Autodesk Inventor part; units mm, degrees
(part 15 of 16)
  spline S109 degree 3 poles (-20.4235, 24.8999) (-20.3314, 25.0779) (-20.2053, 25.3055) (-20.0401, 25.5749) (-19.9493, 25.7161) (-19.8616, 25.8465) (-19.7774, 25.9661) (-19.6971, 26.0752) (-19.6212, 26.174) (-19.55, 26.2628) (-19.4839, 26.3417) (-19.4233, 26.411) (-19.3686, 26.4711) (-19.3201, 26.5222) (-19.2781, 26.5645) (-19.2306, 26.6108) (-19.1862, 26.6499) (-19.1456, 26.6873) (-19.119, 26.7128) (-19.0934, 26.7382) (-19.0688, 26.7635) (-19.0454, 26.7887) (-19.0229, 26.8139) (-19.0014, 26.8391) (-18.9809, 26.8643) (-18.9614, 26.8898) (-18.9428, 26.9154) (-18.925, 26.9415) (-18.9082, 26.9681) (-18.8922, 26.9953) (-18.8771, 27.0236) (-18.863, 27.0531) (-18.8498, 27.0842) (-18.8379, 27.1174) (-18.8274, 27.1531) (-18.8189, 27.192) (-18.813, 27.2347) (-18.8107, 27.2815) (-18.8136, 27.3328) (-18.8231, 27.3881) (-18.8411, 27.4459) (-18.8673, 27.5015) (-18.9487, 27.622) (-19.0935, 27.7983) (-19.2204, 27.9879) (-19.3121, 28.1007) (-19.3578, 28.1419) (-19.4079, 28.1759) (-19.458, 28.201) (-19.5063, 28.2185) (-19.5518, 28.2299) (-19.5943, 28.2366) (-19.634, 28.2397) (-19.6713, 28.24) (-19.7065, 28.2382) (-19.7401, 28.2347) (-19.7724, 28.2296) (-19.8038, 28.2234) (-19.8346, 28.216) (-19.8649, 28.2076) (-19.8949, 28.1981) (-19.9249, 28.1877) (-19.9549, 28.1764) (-19.985, 28.1641) (-20.0153, 28.1508) (-20.046, 28.1366) (-20.0769, 28.1214) (-20.1082, 28.1053) (-20.1399, 28.0881) (-20.172, 28.07) (-20.2196, 28.042) (-20.2698, 28.0108) (-20.3279, 27.9787) (-20.3806, 27.9507) (-20.4435, 27.9191) (-20.5168, 27.8841) (-20.6008, 27.8462) (-20.6954, 27.8058) (-20.801, 27.7633) (-20.9175, 27.7192) (-21.0452, 27.674) (-21.1841, 27.628) (-21.3342, 27.5818) (-21.4957, 27.5358) (-21.8014, 27.4556) (-22.0557, 27.4007) (-22.2528, 27.3641) knots 0 0 0 0 0.085622 0.111078 0.134991 0.157361 0.178189 0.197474 0.215216 0.231415 0.246072 0.259186 0.270757 0.280785 0.28927 0.296213 0.309142 0.314525 0.319779 0.32491 0.329923 0.334826 0.339627 0.344336 0.348964 0.353525 0.358035 0.362514 0.366985 0.371475 0.37602 0.380661 0.385447 0.39044 0.395711 0.401345 0.407436 0.41408 0.421363 0.429333 0.437971 0.447155 0.455484 0.5 0.544516 0.552845 0.562029 0.570667 0.578637 0.58592 0.592564 0.598655 0.604289 0.60956 0.614553 0.619339 0.62398 0.628525 0.633015 0.637486 0.641965 0.646475 0.651036 0.655664 0.660373 0.665174 0.670077 0.67509 0.680221 0.685475 0.690858 0.703787 0.71073 0.719215 0.729243 0.740814 0.753928 0.768585 0.784784 0.802526 0.821811 0.842639 0.865009 0.888922 0.914378 1 1 1 1
  arc A314 (-20.4235, 24.8999) -> (-19.6884, 24.0568) centre (0.0409, 42.0024) ccw
  spline S110 degree 3 poles (-17.4962, 21.9091) (-17.4331, 22.0994) (-17.3441, 22.3438) (-17.223, 22.6357) (-17.1554, 22.7895) (-17.0892, 22.932) (-17.0247, 23.0633) (-16.9626, 23.1836) (-16.903, 23.2931) (-16.8466, 23.3918) (-16.7937, 23.4801) (-16.7447, 23.5581) (-16.7, 23.626) (-16.6601, 23.684) (-16.6253, 23.7324) (-16.5855, 23.7856) (-16.5478, 23.8311) (-16.5136, 23.8744) (-16.4912, 23.9038) (-16.4699, 23.9329) (-16.4497, 23.9617) (-16.4304, 23.9902) (-16.4122, 24.0186) (-16.3949, 24.0469) (-16.3786, 24.075) (-16.3633, 24.1032) (-16.3489, 24.1315) (-16.3355, 24.16) (-16.323, 24.1889) (-16.3115, 24.2183) (-16.301, 24.2486) (-16.2916, 24.2799) (-16.2835, 24.3127) (-16.2769, 24.3473) (-16.2722, 24.3843) (-16.2698, 24.424) (-16.2707, 24.4671) (-16.2758, 24.5137) (-16.2866, 24.5639) (-16.3047, 24.617) (-16.3315, 24.6713) (-16.3661, 24.7221) (-16.4653, 24.8284) (-16.636, 24.9798) (-16.7909, 25.1473) (-16.8991, 25.2444) (-16.9507, 25.2779) (-17.0055, 25.3036) (-17.0589, 25.3206) (-17.1094, 25.3304) (-17.1561, 25.3345) (-17.1992, 25.3345) (-17.2389, 25.3313) (-17.2757, 25.3258) (-17.3102, 25.3185) (-17.3428, 25.3097) (-17.3739, 25.2997) (-17.404, 25.2886) (-17.4332, 25.2765) (-17.4618, 25.2634) (-17.49, 25.2494) (-17.518, 25.2345) (-17.5459, 25.2185) (-17.5737, 25.2017) (-17.6016, 25.1838) (-17.6296, 25.165) (-17.6577, 25.1452) (-17.6861, 25.1243) (-17.7148, 25.1024) (-17.7437, 25.0795) (-17.7863, 25.0444) (-17.831, 25.0058) (-17.8834, 24.9649) (-17.931, 24.9291) (-17.9882, 24.888) (-18.0551, 24.842) (-18.1321, 24.7914) (-18.2193, 24.7367) (-18.3169, 24.6782) (-18.4251, 24.6165) (-18.5441, 24.5518) (-18.6741, 24.4847) (-18.8152, 24.4156) (-18.9675, 24.3448) (-19.2569, 24.2178) (-19.4995, 24.1238) (-19.6884, 24.0568) knots 0 0 0 0 0.085622 0.111078 0.134991 0.157361 0.178189 0.197474 0.215216 0.231415 0.246072 0.259186 0.270757 0.280785 0.28927 0.296213 0.309142 0.314525 0.319779 0.32491 0.329923 0.334826 0.339627 0.344336 0.348964 0.353525 0.358035 0.362514 0.366985 0.371475 0.37602 0.380661 0.385447 0.39044 0.395711 0.401345 0.407436 0.41408 0.421363 0.429333 0.437971 0.447155 0.455484 0.5 0.544516 0.552845 0.562029 0.570667 0.578637 0.58592 0.592564 0.598655 0.604289 0.60956 0.614553 0.619339 0.62398 0.628525 0.633015 0.637486 0.641965 0.646475 0.651036 0.655664 0.660373 0.665174 0.670077 0.67509 0.680221 0.685475 0.690858 0.703787 0.71073 0.719215 0.729243 0.740814 0.753928 0.768585 0.784784 0.802526 0.821811 0.842639 0.865009 0.888922 0.914378 1 1 1 1
  arc A315 (-17.4962, 21.9091) -> (-16.6382, 21.1914) centre (0.0409, 42.0024) ccw
  spline S111 degree 3 poles (-14.137, 19.4131) (-14.1044, 19.6109) (-14.0548, 19.8663) (-13.9809, 20.1735) (-13.9381, 20.3359) (-13.895, 20.487) (-13.8519, 20.6268) (-13.8093, 20.7554) (-13.7676, 20.8728) (-13.7273, 20.9792) (-13.6889, 21.0747) (-13.6527, 21.1594) (-13.6192, 21.2334) (-13.5889, 21.297) (-13.562, 21.3502) (-13.5311, 21.4089) (-13.5009, 21.4598) (-13.4739, 21.5079) (-13.4565, 21.5404) (-13.44, 21.5725) (-13.4245, 21.6041) (-13.4099, 21.6353) (-13.3963, 21.6662) (-13.3837, 21.6968) (-13.372, 21.7272) (-13.3613, 21.7574) (-13.3515, 21.7876) (-13.3427, 21.8178) (-13.3349, 21.8483) (-13.3281, 21.8792) (-13.3225, 21.9107) (-13.3182, 21.9431) (-13.3153, 21.9768) (-13.3142, 22.012) (-13.3153, 22.0493) (-13.3192, 22.0889) (-13.3267, 22.1313) (-13.3391, 22.1765) (-13.3576, 22.2244) (-13.3837, 22.2741) (-13.4187, 22.3235) (-13.4608, 22.3683) (-13.5755, 22.4577) (-13.7677, 22.5806) (-13.9469, 22.7218) (-14.069, 22.8007) (-14.1252, 22.8258) (-14.1834, 22.8426) (-14.2388, 22.851) (-14.2901, 22.8527) (-14.337, 22.8495) (-14.3795, 22.8427) (-14.4182, 22.8334) (-14.4537, 22.8222) (-14.4866, 22.8096) (-14.5175, 22.7958) (-14.5467, 22.7811) (-14.5746, 22.7654) (-14.6016, 22.7489) (-14.6278, 22.7315) (-14.6535, 22.7132) (-14.6787, 22.6941) (-14.7038, 22.674) (-14.7286, 22.653) (-14.7533, 22.631) (-14.7781, 22.608) (-14.8028, 22.5841) (-14.8276, 22.559) (-14.8524, 22.5329) (-14.8774, 22.5057) (-14.914, 22.4644) (-14.9521, 22.4192) (-14.9974, 22.3707) (-15.0389, 22.3279) (-15.0889, 22.2784) (-15.1479, 22.2224) (-15.216, 22.1604) (-15.2935, 22.0927) (-15.3808, 22.0197) (-15.478, 21.9418) (-15.5855, 21.8593) (-15.7033, 21.7727) (-15.8319, 21.6823) (-15.9712, 21.5886) (-16.2372, 21.4179) (-16.4621, 21.2871) (-16.6382, 21.1914) knots 0 0 0 0 0.085622 0.111078 0.134991 0.157361 0.178189 0.197474 0.215216 0.231415 0.246072 0.259186 0.270757 0.280785 0.28927 0.296213 0.309142 0.314525 0.319779 0.32491 0.329923 0.334826 0.339627 0.344336 0.348964 0.353525 0.358035 0.362514 0.366985 0.371475 0.37602 0.380661 0.385447 0.39044 0.395711 0.401345 0.407436 0.41408 0.421363 0.429333 0.437971 0.447155 0.455484 0.5 0.544516 0.552845 0.562029 0.570667 0.578637 0.58592 0.592564 0.598655 0.604289 0.60956 0.614553 0.619339 0.62398 0.628525 0.633015 0.637486 0.641965 0.646475 0.651036 0.655664 0.660373 0.665174 0.670077 0.67509 0.680221 0.685475 0.690858 0.703787 0.71073 0.719215 0.729243 0.740814 0.753928 0.768585 0.784784 0.802526 0.821811 0.842639 0.865009 0.888922 0.914378 1 1 1 1
  arc A316 (-14.137, 19.4131) -> (-13.1773, 18.8385) centre (0.0409, 42.0024) ccw
  spline S112 degree 3 poles (-10.4287, 17.4733) (-10.4274, 17.6737) (-10.4184, 17.9337) (-10.3934, 18.2488) (-10.3767, 18.4159) (-10.3577, 18.5718) (-10.337, 18.7166) (-10.315, 18.8503) (-10.2922, 18.9728) (-10.2691, 19.0842) (-10.246, 19.1845) (-10.2235, 19.2738) (-10.2021, 19.3522) (-10.182, 19.4197) (-10.1638, 19.4765) (-10.1425, 19.5393) (-10.1206, 19.5943) (-10.1015, 19.646) (-10.0893, 19.6809) (-10.0781, 19.7151) (-10.0677, 19.7488) (-10.0582, 19.7819) (-10.0496, 19.8145) (-10.0419, 19.8467) (-10.0351, 19.8785) (-10.0293, 19.9101) (-10.0243, 19.9414) (-10.0203, 19.9727) (-10.0174, 20.004) (-10.0156, 20.0356) (-10.0149, 20.0676) (-10.0157, 20.1003) (-10.0182, 20.134) (-10.0226, 20.1689) (-10.0295, 20.2055) (-10.0395, 20.2441) (-10.0536, 20.2847) (-10.0729, 20.3275) (-10.0987, 20.372) (-10.1323, 20.4169) (-10.1745, 20.4602) (-10.2232, 20.4979) (-10.3504, 20.5682) (-10.5595, 20.6596) (-10.7586, 20.771) (-10.8915, 20.8298) (-10.9509, 20.8458) (-11.011, 20.8533) (-11.0671, 20.8529) (-11.118, 20.8466) (-11.1638, 20.8361) (-11.2047, 20.8228) (-11.2415, 20.8075) (-11.2748, 20.7909) (-11.3053, 20.7733) (-11.3337, 20.7549) (-11.3602, 20.7357) (-11.3853, 20.7159) (-11.4094, 20.6953) (-11.4325, 20.6741) (-11.4551, 20.652) (-11.477, 20.6291) (-11.4986, 20.6054) (-11.5199, 20.5808) (-11.5409, 20.5552) (-11.5617, 20.5286) (-11.5823, 20.5011) (-11.6029, 20.4725) (-11.6234, 20.4428) (-11.6438, 20.412) (-11.6734, 20.3655) (-11.704, 20.3149) (-11.7412, 20.2599) (-11.7754, 20.2111) (-11.8171, 20.1544) (-11.8666, 20.0899) (-11.9242, 20.018) (-11.9902, 19.939) (-12.065, 19.8533) (-12.1488, 19.7611) (-12.242, 19.6628) (-12.3449, 19.5588) (-12.4577, 19.4495) (-12.5807, 19.3351) (-12.8166, 19.1249) (-13.0183, 18.9605) (-13.1773, 18.8385) knots 0 0 0 0 0.085622 0.111078 0.134991 0.157361 0.178189 0.197474 0.215216 0.231415 0.246072 0.259186 0.270757 0.280785 0.28927 0.296213 0.309142 0.314525 0.319779 0.32491 0.329923 0.334826 0.339627 0.344336 0.348964 0.353525 0.358035 0.362514 0.366985 0.371475 0.37602 0.380661 0.385447 0.39044 0.395711 0.401345 0.407436 0.41408 0.421363 0.429333 0.437971 0.447155 0.455484 0.5 0.544516 0.552845 0.562029 0.570667 0.578637 0.58592 0.592564 0.598655 0.604289 0.60956 0.614553 0.619339 0.62398 0.628525 0.633015 0.637486 0.641965 0.646475 0.651036 0.655664 0.660373 0.665174 0.670077 0.67509 0.680221 0.685475 0.690858 0.703787 0.71073 0.719215 0.729243 0.740814 0.753928 0.768585 0.784784 0.802526 0.821811 0.842639 0.865009 0.888922 0.914378 1 1 1 1
  arc A317 (-10.4287, 17.4733) -> (-9.3909, 17.0559) centre (0.0409, 42.0024) ccw
  spline S113 degree 3 poles (-6.4626, 16.1375) (-6.4927, 16.3356) (-6.5245, 16.5939) (-6.5491, 16.9089) (-6.5587, 17.0766) (-6.5643, 17.2336) (-6.5665, 17.3799) (-6.5657, 17.5153) (-6.5624, 17.6399) (-6.557, 17.7535) (-6.5499, 17.8562) (-6.5416, 17.9479) (-6.5327, 18.0287) (-6.5235, 18.0985) (-6.5144, 18.1574) (-6.5031, 18.2228) (-6.4901, 18.2805) (-6.4793, 18.3346) (-6.4728, 18.371) (-6.467, 18.4065) (-6.462, 18.4414) (-6.4578, 18.4756) (-6.4545, 18.5092) (-6.4519, 18.5422) (-6.4502, 18.5747) (-6.4493, 18.6067) (-6.4493, 18.6385) (-6.4503, 18.67) (-6.4523, 18.7014) (-6.4554, 18.7328) (-6.4598, 18.7646) (-6.4657, 18.7967) (-6.4733, 18.8296) (-6.4832, 18.8635) (-6.4957, 18.8985) (-6.5117, 18.935) (-6.532, 18.973) (-6.5577, 19.0122) (-6.5901, 19.0521) (-6.6303, 19.0912) (-6.6788, 19.1274) (-6.7327, 19.157) (-6.8694, 19.2066) (-7.0902, 19.2641) (-7.3043, 19.3429) (-7.4448, 19.3803) (-7.506, 19.3868) (-7.5665, 19.3848) (-7.6218, 19.3756) (-7.6712, 19.3614) (-7.7147, 19.3439) (-7.753, 19.3243) (-7.787, 19.3035) (-7.8173, 19.2819) (-7.8447, 19.2597) (-7.8698, 19.2371) (-7.893, 19.214) (-7.9147, 19.1905) (-7.9352, 19.1665) (-7.9548, 19.1418) (-7.9736, 19.1165) (-7.9917, 19.0905) (-8.0093, 19.0637) (-8.0264, 19.036) (-8.0432, 19.0074) (-8.0596, 18.978) (-8.0757, 18.9475) (-8.0915, 18.916) (-8.1071, 18.8835) (-8.1224, 18.85) (-8.1445, 18.7994) (-8.1668, 18.7446) (-8.1949, 18.6845) (-8.2211, 18.6309) (-8.2534, 18.5683) (-8.2921, 18.4969) (-8.3377, 18.4169) (-8.3906, 18.3286) (-8.451, 18.2322) (-8.5194, 18.128) (-8.5961, 18.0164) (-8.6814, 17.8976) (-8.7757, 17.7719) (-8.8794, 17.6397) (-9.0795, 17.3952) (-9.253, 17.2013) (-9.3909, 17.0559) knots 0 0 0 0 0.085622 0.111078 0.134991 0.157361 0.178189 0.197474 0.215216 0.231415 0.246072 0.259186 0.270757 0.280785 0.28927 0.296213 0.309142 0.314525 0.319779 0.32491 0.329923 0.334826 0.339627 0.344336 0.348964 0.353525 0.358035 0.362514 0.366985 0.371475 0.37602 0.380661 0.385447 0.39044 0.395711 0.401345 0.407436 0.41408 0.421363 0.429333 0.437971 0.447155 0.455484 0.5 0.544516 0.552845 0.562029 0.570667 0.578637 0.58592 0.592564 0.598655 0.604289 0.60956 0.614553 0.619339 0.62398 0.628525 0.633015 0.637486 0.641965 0.646475 0.651036 0.655664 0.660373 0.665174 0.670077 0.67509 0.680221 0.685475 0.690858 0.703787 0.71073 0.719215 0.729243 0.740814 0.753928 0.768585 0.784784 0.802526 0.821811 0.842639 0.865009 0.888922 0.914378 1 1 1 1
  arc A318 (-6.4626, 16.1375) -> (-5.3723, 15.8875) centre (0.0409, 42.0024) ccw
  spline S114 degree 3 poles (-2.3363, 15.4385) (-2.3971, 15.6296) (-2.4689, 15.8796) (-2.5425, 16.187) (-2.5782, 16.3511) (-2.6083, 16.5053) (-2.6334, 16.6494) (-2.6538, 16.7833) (-2.67, 16.9068) (-2.6824, 17.0199) (-2.6914, 17.1225) (-2.6977, 17.2143) (-2.7014, 17.2955) (-2.7032, 17.3659) (-2.7035, 17.4255) (-2.7026, 17.4919) (-2.6988, 17.5509) (-2.6966, 17.606) (-2.6958, 17.6429) (-2.6956, 17.679) (-2.6962, 17.7142) (-2.6974, 17.7486) (-2.6993, 17.7823) (-2.702, 17.8153) (-2.7053, 17.8477) (-2.7095, 17.8795) (-2.7145, 17.9108) (-2.7204, 17.9418) (-2.7272, 17.9725) (-2.7352, 18.0031) (-2.7445, 18.0337) (-2.7554, 18.0646) (-2.7681, 18.0959) (-2.7831, 18.1278) (-2.801, 18.1604) (-2.8225, 18.194) (-2.8484, 18.2283) (-2.88, 18.263) (-2.9183, 18.2973) (-2.9641, 18.3297) (-3.0177, 18.3578) (-3.0755, 18.3786) (-3.2183, 18.4062) (-3.4454, 18.4284) (-3.6691, 18.4729) (-3.8138, 18.4878) (-3.8752, 18.4846) (-3.9346, 18.4732) (-3.9879, 18.4555) (-4.0344, 18.4338) (-4.0746, 18.4096) (-4.1094, 18.3843) (-4.1397, 18.3584) (-4.1663, 18.3323) (-4.1899, 18.3061) (-4.2111, 18.2799) (-4.2304, 18.2535) (-4.2482, 18.2268) (-4.2647, 18.1999) (-4.2802, 18.1725) (-4.2948, 18.1445) (-4.3086, 18.116) (-4.3218, 18.0867) (-4.3344, 18.0567) (-4.3465, 18.0259) (-4.358, 17.9942) (-4.3692, 17.9616) (-4.3799, 17.9281) (-4.3902, 17.8935) (-4.4001, 17.858) (-4.4139, 17.8046) (-4.4274, 17.747) (-4.4458, 17.6832) (-4.4632, 17.6262) (-4.4854, 17.5593) (-4.5125, 17.4827) (-4.545, 17.3966) (-4.5834, 17.3011) (-4.628, 17.1964) (-4.6792, 17.0828) (-4.7375, 16.9606) (-4.8032, 16.8299) (-4.8767, 16.691) (-4.9584, 16.5442) (-5.1178, 16.2714) (-5.2588, 16.0528) (-5.3723, 15.8875) knots 0 0 0 0 0.085622 0.111078 0.134991 0.157361 0.178189 0.197474 0.215216 0.231415 0.246072 0.259186 0.270757 0.280785 0.28927 0.296213 0.309142 0.314525 0.319779 0.32491 0.329923 0.334826 0.339627 0.344336 0.348964 0.353525 0.358035 0.362514 0.366985 0.371475 0.37602 0.380661 0.385447 0.39044 0.395711 0.401345 0.407436 0.41408 0.421363 0.429333 0.437971 0.447155 0.455484 0.5 0.544516 0.552845 0.562029 0.570667 0.578637 0.58592 0.592564 0.598655 0.604289 0.60956 0.614553 0.619339 0.62398 0.628525 0.633015 0.637486 0.641965 0.646475 0.651036 0.655664 0.660373 0.665174 0.670077 0.67509 0.680221 0.685475 0.690858 0.703787 0.71073 0.719215 0.729243 0.740814 0.753928 0.768585 0.784784 0.802526 0.821811 0.842639 0.865009 0.888922 0.914378 1 1 1 1
  arc A319 (-2.3363, 15.4385) -> (-1.2204, 15.3622) centre (0.0409, 42.0024) ccw
  spline S115 degree 3 poles (1.8484, 15.3937) (1.7585, 15.5729) (1.6485, 15.8086) (1.5278, 16.1007) (1.4668, 16.2572) (1.4129, 16.4048) (1.3656, 16.5432) (1.3245, 16.6722) (1.2892, 16.7917) (1.2593, 16.9015) (1.2343, 17.0013) (1.2138, 17.0911) (1.1973, 17.1707) (1.1845, 17.24) (1.175, 17.2988) (1.1655, 17.3645) (1.16, 17.4234) (1.1535, 17.4782) (1.1486, 17.5147) (1.1431, 17.5504) (1.137, 17.5851) (1.1304, 17.6189) (1.1233, 17.6519) (1.1155, 17.684) (1.1071, 17.7155) (1.098, 17.7462) (1.0882, 17.7764) (1.0775, 17.806) (1.066, 17.8353) (1.0533, 17.8643) (1.0393, 17.8931) (1.0237, 17.9219) (1.0063, 17.9508) (0.9865, 17.9799) (0.9637, 18.0094) (0.9372, 18.0392) (0.9062, 18.069) (0.8696, 18.0984) (0.8265, 18.1263) (0.7762, 18.151) (0.7188, 18.1704) (0.6584, 18.1819) (0.5131, 18.1869) (0.2853, 18.1733) (0.0574, 18.1822) (-0.0878, 18.1743) (-0.148, 18.1616) (-0.2049, 18.141) (-0.2547, 18.1152) (-0.2973, 18.0864) (-0.3333, 18.0563) (-0.3637, 18.0258) (-0.3895, 17.9955) (-0.4117, 17.9656) (-0.4309, 17.936) (-0.4477, 17.9068) (-0.4627, 17.8777) (-0.4761, 17.8486) (-0.4882, 17.8194) (-0.4992, 17.7899) (-0.5092, 17.76) (-0.5184, 17.7296) (-0.5268, 17.6987) (-0.5346, 17.6671) (-0.5417, 17.6348) (-0.5482, 17.6017) (-0.5541, 17.5677) (-0.5594, 17.5329) (-0.5642, 17.4972) (-0.5684, 17.4605) (-0.5737, 17.4056) (-0.578, 17.3466) (-0.5862, 17.2807) (-0.5945, 17.2217) (-0.6059, 17.1522) (-0.6207, 17.0723) (-0.6393, 16.9821) (-0.6623, 16.8818) (-0.69, 16.7714) (-0.7229, 16.6512) (-0.7613, 16.5214) (-0.8057, 16.382) (-0.8566, 16.2333) (-0.9143, 16.0756) (-1.0291, 15.7812) (-1.1342, 15.5432) (-1.2204, 15.3622) knots 0 0 0 0 0.085622 0.111078 0.134991 0.157361 0.178189 0.197474 0.215216 0.231415 0.246072 0.259186 0.270757 0.280785 0.28927 0.296213 0.309142 0.314525 0.319779 0.32491 0.329923 0.334826 0.339627 0.344336 0.348964 0.353525 0.358035 0.362514 0.366985 0.371475 0.37602 0.380661 0.385447 0.39044 0.395711 0.401345 0.407436 0.41408 0.421363 0.429333 0.437971 0.447155 0.455484 0.5 0.544516 0.552845 0.562029 0.570667 0.578637 0.58592 0.592564 0.598655 0.604289 0.60956 0.614553 0.619339 0.62398 0.628525 0.633015 0.637486 0.641965 0.646475 0.651036 0.655664 0.660373 0.665174 0.670077 0.67509 0.680221 0.685475 0.690858 0.703787 0.71073 0.719215 0.729243 0.740814 0.753928 0.768585 0.784784 0.802526 0.821811 0.842639 0.865009 0.888922 0.914378 1 1 1 1
  arc A320 (1.8484, 15.3937) -> (2.9626, 15.4929) centre (0.0409, 42.0024) ccw
  spline S116 degree 3 poles (5.9887, 16.0041) (5.8719, 16.1669) (5.7263, 16.3826) (5.5614, 16.6522) (5.4767, 16.7972) (5.4004, 16.9345) (5.332, 17.0638) (5.2713, 17.1849) (5.2177, 17.2974) (5.1709, 17.4011) (5.1306, 17.4958) (5.0963, 17.5813) (5.0676, 17.6573) (5.0441, 17.7237) (5.0255, 17.7803) (5.0058, 17.8437) (4.9912, 17.901) (4.9763, 17.9541) (4.9656, 17.9895) (4.9546, 18.0238) (4.9432, 18.0572) (4.9314, 18.0895) (4.9192, 18.121) (4.9065, 18.1515) (4.8933, 18.1813) (4.8795, 18.2102) (4.8651, 18.2385) (4.8499, 18.2661) (4.8339, 18.2932) (4.8168, 18.3198) (4.7985, 18.3461) (4.7786, 18.3721) (4.7569, 18.3979) (4.7328, 18.4236) (4.7057, 18.4491) (4.6749, 18.4744) (4.6396, 18.499) (4.5988, 18.5223) (4.5518, 18.5431) (4.4983, 18.5597) (4.4386, 18.5699) (4.3771, 18.5718) (4.2328, 18.5539) (4.01, 18.5049) (3.7835, 18.478) (3.6413, 18.4475) (3.5839, 18.4255) (3.5309, 18.3963) (3.4857, 18.363) (3.4482, 18.328) (3.4173, 18.2926) (3.3921, 18.2577) (3.3713, 18.2237) (3.3541, 18.1907) (3.3397, 18.1585) (3.3277, 18.127) (3.3175, 18.0959) (3.3088, 18.0651) (3.3014, 18.0343) (3.2952, 18.0035) (3.2899, 17.9724) (3.2856, 17.941) (3.2821, 17.9091) (3.2794, 17.8767) (3.2774, 17.8436) (3.2762, 17.8099) (3.2757, 17.7755) (3.2758, 17.7402) (3.2767, 17.7042) (3.2783, 17.6673) (3.2816, 17.6123) (3.2866, 17.5533) (3.2889, 17.487) (3.2899, 17.4274) (3.2895, 17.357) (3.2874, 17.2757) (3.2831, 17.1837) (3.2761, 17.081) (3.266, 16.9677) (3.2523, 16.8439) (3.2347, 16.7096) (3.2126, 16.565) (3.1856, 16.4102) (3.1533, 16.2454) (3.086, 15.9366) (3.0194, 15.6851) (2.9626, 15.4929) knots 0 0 0 0 0.085622 0.111078 0.134991 0.157361 0.178189 0.197474 0.215216 0.231415 0.246072 0.259186 0.270757 0.280785 0.28927 0.296213 0.309142 0.314525 0.319779 0.32491 0.329923 0.334826 0.339627 0.344336 0.348964 0.353525 0.358035 0.362514 0.366985 0.371475 0.37602 0.380661 0.385447 0.39044 0.395711 0.401345 0.407436 0.41408 0.421363 0.429333 0.437971 0.447155 0.455484 0.5 0.544516 0.552845 0.562029 0.570667 0.578637 0.58592 0.592564 0.598655 0.604289 0.60956 0.614553 0.619339 0.62398 0.628525 0.633015 0.637486 0.641965 0.646475 0.651036 0.655664 0.660373 0.665174 0.670077 0.67509 0.680221 0.685475 0.690858 0.703787 0.71073 0.719215 0.729243 0.740814 0.753928 0.768585 0.784784 0.802526 0.821811 0.842639 0.865009 0.888922 0.914378 1 1 1 1
  arc A321 (5.9887, 16.0041) -> (7.0736, 16.2763) centre (0.0409, 42.0024) ccw
  spline S117 degree 3 poles (9.9825, 17.2546) (9.8416, 17.3972) (9.6642, 17.5874) (9.4591, 17.8278) (9.3528, 17.9579) (9.2559, 18.0816) (9.1681, 18.1986) (9.0892, 18.3086) (9.0187, 18.4114) (8.9563, 18.5065) (8.9016, 18.5937) (8.8544, 18.6728) (8.8142, 18.7434) (8.7806, 18.8053) (8.7533, 18.8583) (8.724, 18.9179) (8.7005, 18.9722) (8.6775, 19.0223) (8.6614, 19.0555) (8.6452, 19.0877) (8.6287, 19.1189) (8.612, 19.149) (8.595, 19.1781) (8.5777, 19.2063) (8.56, 19.2336) (8.5418, 19.2601) (8.5232, 19.2857) (8.5039, 19.3106) (8.4838, 19.3349) (8.4628, 19.3585) (8.4406, 19.3816) (8.4169, 19.4042) (8.3914, 19.4263) (8.3635, 19.4479) (8.3328, 19.4689) (8.2984, 19.489) (8.2597, 19.5078) (8.2158, 19.5244) (8.1662, 19.5376) (8.1107, 19.5456) (8.0501, 19.5464) (7.9891, 19.5386) (7.8494, 19.4984) (7.637, 19.4151) (7.4174, 19.3531) (7.2818, 19.3007) (7.2285, 19.27) (7.1807, 19.2329) (7.1413, 19.1929) (7.1097, 19.1524) (7.0848, 19.1127) (7.0653, 19.0743) (7.0501, 19.0375) (7.0383, 19.0022) (7.0291, 18.9681) (7.0221, 18.9351) (7.0169, 18.9028) (7.0132, 18.871) (7.0107, 18.8395) (7.0093, 18.808) (7.009, 18.7765) (7.0097, 18.7448) (7.0112, 18.7128) (7.0136, 18.6803) (7.0168, 18.6474) (7.0209, 18.6139) (7.0258, 18.5798) (7.0315, 18.545) (7.038, 18.5096) (7.0453, 18.4734) (7.0572, 18.4195) (7.0713, 18.3621) (7.084, 18.2969) (7.0942, 18.2382) (7.1049, 18.1686) (7.1155, 18.088) (7.1256, 17.9965) (7.1348, 17.894) (7.1426, 17.7805) (7.1485, 17.656) (7.152, 17.5206) (7.1528, 17.3743) (7.1504, 17.2172) (7.1443, 17.0494) (7.1261, 16.7339) (7.0997, 16.4751) (7.0736, 16.2763) knots 0 0 0 0 0.085622 0.111078 0.134991 0.157361 0.178189 0.197474 0.215216 0.231415 0.246072 0.259186 0.270757 0.280785 0.28927 0.296213 0.309142 0.314525 0.319779 0.32491 0.329923 0.334826 0.339627 0.344336 0.348964 0.353525 0.358035 0.362514 0.366985 0.371475 0.37602 0.380661 0.385447 0.39044 0.395711 0.401345 0.407436 0.41408 0.421363 0.429333 0.437971 0.447155 0.455484 0.5 0.544516 0.552845 0.562029 0.570667 0.578637 0.58592 0.592564 0.598655 0.604289 0.60956 0.614553 0.619339 0.62398 0.628525 0.633015 0.637486 0.641965 0.646475 0.651036 0.655664 0.660373 0.665174 0.670077 0.67509 0.680221 0.685475 0.690858 0.703787 0.71073 0.719215 0.729243 0.740814 0.753928 0.768585 0.784784 0.802526 0.821811 0.842639 0.865009 0.888922 0.914378 1 1 1 1
  arc A322 (9.9825, 17.2546) -> (11.0115, 17.6932) centre (0.0409, 42.0024) ccw
  spline S118 degree 3 poles (13.7315, 19.1145) (13.5701, 19.2333) (13.365, 19.3934) (13.1248, 19.5988) (12.9995, 19.7106) (12.8845, 19.8176) (12.7795, 19.9195) (12.6843, 20.0158) (12.5986, 20.1062) (12.5221, 20.1904) (12.4544, 20.2681) (12.3954, 20.3388) (12.3446, 20.4022) (12.3018, 20.4581) (12.2666, 20.5062) (12.2283, 20.5604) (12.1966, 20.6104) (12.166, 20.6563) (12.145, 20.6866) (12.1239, 20.7158) (12.1028, 20.744) (12.0815, 20.7712) (12.0602, 20.7973) (12.0387, 20.8224) (12.0169, 20.8466) (11.9949, 20.8699) (11.9724, 20.8923) (11.9495, 20.9139) (11.9259, 20.9347) (11.9014, 20.9548) (11.8759, 20.9741) (11.8489, 20.9927) (11.8203, 21.0105) (11.7894, 21.0275) (11.7557, 21.0434) (11.7186, 21.0579) (11.6774, 21.0704) (11.6315, 21.08) (11.5804, 21.0852) (11.5243, 21.0845) (11.4644, 21.0757) (11.4054, 21.0585) (11.2736, 20.997) (11.0769, 20.8815) (10.8697, 20.7859) (10.7439, 20.7129) (10.6961, 20.6743) (10.6547, 20.6301) (10.6221, 20.5845) (10.5972, 20.5396) (10.5788, 20.4964) (10.5656, 20.4554) (10.5563, 20.4167) (10.5502, 20.38) (10.5464, 20.3449) (10.5447, 20.3112) (10.5446, 20.2785) (10.5459, 20.2465) (10.5484, 20.215) (10.552, 20.1837) (10.5566, 20.1525) (10.5622, 20.1213) (10.5687, 20.0899) (10.5761, 20.0582) (10.5845, 20.0262) (10.5937, 19.9937) (10.6039, 19.9608) (10.6149, 19.9274) (10.6269, 19.8934) (10.6398, 19.8588) (10.66, 19.8074) (10.6829, 19.7529) (10.7056, 19.6905) (10.7249, 19.6342) (10.7463, 19.5671) (10.7694, 19.4892) (10.7938, 19.4003) (10.8189, 19.3005) (10.8443, 19.1896) (10.8696, 19.0676) (10.8943, 18.9344) (10.918, 18.7901) (10.9401, 18.6345) (10.9603, 18.4678) (10.9918, 18.1534) (11.0061, 17.8936) (11.0115, 17.6932) knots 0 0 0 0 0.085622 0.111078 0.134991 0.157361 0.178189 0.197474 0.215216 0.231415 0.246072 0.259186 0.270757 0.280785 0.28927 0.296213 0.309142 0.314525 0.319779 0.32491 0.329923 0.334826 0.339627 0.344336 0.348964 0.353525 0.358035 0.362514 0.366985 0.371475 0.37602 0.380661 0.385447 0.39044 0.395711 0.401345 0.407436 0.41408 0.421363 0.429333 0.437971 0.447155 0.455484 0.5 0.544516 0.552845 0.562029 0.570667 0.578637 0.58592 0.592564 0.598655 0.604289 0.60956 0.614553 0.619339 0.62398 0.628525 0.633015 0.637486 0.641965 0.646475 0.651036 0.655664 0.660373 0.665174 0.670077 0.67509 0.680221 0.685475 0.690858 0.703787 0.71073 0.719215 0.729243 0.740814 0.753928 0.768585 0.784784 0.802526 0.821811 0.842639 0.865009 0.888922 0.914378 1 1 1 1
  arc A323 (13.7315, 19.1145) -> (14.6792, 19.7087) centre (0.0409, 42.0024) ccw
  spline S119 degree 3 poles (17.1434, 21.5379) (16.9654, 21.63) (16.7378, 21.7561) (16.4684, 21.9214) (16.3272, 22.0122) (16.1968, 22.0999) (16.0772, 22.1841) (15.9681, 22.2644) (15.8693, 22.3403) (15.7805, 22.4115) (15.7016, 22.4776) (15.6322, 22.5381) (15.5722, 22.5929) (15.5211, 22.6414) (15.4788, 22.6833) (15.4325, 22.7309) (15.3934, 22.7753) (15.356, 22.8159) (15.3305, 22.8425) (15.3051, 22.8681) (15.2798, 22.8926) (15.2546, 22.9161) (15.2294, 22.9386) (15.2042, 22.96) (15.179, 22.9805) (15.1535, 23.0001) (15.1279, 23.0187) (15.1018, 23.0365) (15.0752, 23.0533) (15.0479, 23.0693) (15.0197, 23.0844) (14.9902, 23.0985) (14.9591, 23.1116) (14.9259, 23.1236) (14.8902, 23.134) (14.8513, 23.1426) (14.8086, 23.1485) (14.7618, 23.1507) (14.7105, 23.1479) (14.6552, 23.1384) (14.5974, 23.1204) (14.5418, 23.0942) (14.4213, 23.0128) (14.245, 22.8679) (14.0554, 22.7411) (13.9426, 22.6494) (13.9014, 22.6037) (13.8674, 22.5536) (13.8423, 22.5035) (13.8248, 22.4552) (13.8134, 22.4097) (13.8067, 22.3671) (13.8036, 22.3274) (13.8033, 22.2902) (13.8051, 22.255) (13.8086, 22.2214) (13.8136, 22.1891) (13.8199, 22.1577) (13.8273, 22.1269) (13.8357, 22.0966) (13.8452, 22.0665) (13.8556, 22.0366) (13.8669, 22.0066) (13.8792, 21.9765) (13.8925, 21.9461) (13.9067, 21.9155) (13.9219, 21.8846) (13.938, 21.8533) (13.9552, 21.8216) (13.9733, 21.7894) (14.0013, 21.7419) (14.0325, 21.6917) (14.0646, 21.6336) (14.0926, 21.5809) (14.1242, 21.518) (14.1592, 21.4446) (14.1971, 21.3607) (14.2375, 21.266) (14.28, 21.1605) (14.3241, 21.0439) (14.3693, 20.9163) (14.4152, 20.7774) (14.4615, 20.6272) (14.5075, 20.4657) (14.5877, 20.1601) (14.6426, 19.9057) (14.6792, 19.7087) knots 0 0 0 0 0.085622 0.111078 0.134991 0.157361 0.178189 0.197474 0.215216 0.231415 0.246072 0.259186 0.270757 0.280785 0.28927 0.296213 0.309142 0.314525 0.319779 0.32491 0.329923 0.334826 0.339627 0.344336 0.348964 0.353525 0.358035 0.362514 0.366985 0.371475 0.37602 0.380661 0.385447 0.39044 0.395711 0.401345 0.407436 0.41408 0.421363 0.429333 0.437971 0.447155 0.455484 0.5 0.544516 0.552845 0.562029 0.570667 0.578637 0.58592 0.592564 0.598655 0.604289 0.60956 0.614553 0.619339 0.62398 0.628525 0.633015 0.637486 0.641965 0.646475 0.651036 0.655664 0.660373 0.665174 0.670077 0.67509 0.680221 0.685475 0.690858 0.703787 0.71073 0.719215 0.729243 0.740814 0.753928 0.768585 0.784784 0.802526 0.821811 0.842639 0.865009 0.888922 0.914378 1 1 1 1
  arc A324 (17.1434, 21.5379) -> (17.9865, 22.2731) centre (0.0409, 42.0024) ccw
  spline S120 degree 3 poles (20.1342, 24.4653) (19.9439, 24.5284) (19.6994, 24.6174) (19.4076, 24.7385) (19.2538, 24.8061) (19.1113, 24.8723) (18.98, 24.9367) (18.8597, 24.9989) (18.7502, 25.0585) (18.6515, 25.1149) (18.5632, 25.1678) (18.4852, 25.2168) (18.4173, 25.2615) (18.3592, 25.3014) (18.3109, 25.3362) (18.2577, 25.3759) (18.2122, 25.4137) (18.1689, 25.4479) (18.1395, 25.4702) (18.1104, 25.4915) (18.0816, 25.5118) (18.053, 25.531) (18.0247, 25.5493) (17.9964, 25.5666) (17.9683, 25.5828) (17.9401, 25.5982) (17.9118, 25.6126) (17.8833, 25.626) (17.8544, 25.6385) (17.825, 25.65) (17.7947, 25.6605) (17.7634, 25.6698) (17.7306, 25.6779) (17.696, 25.6845) (17.659, 25.6893) (17.6193, 25.6916) (17.5762, 25.6908) (17.5296, 25.6857) (17.4794, 25.6749) (17.4263, 25.6568) (17.372, 25.63) (17.3212, 25.5954) (17.2149, 25.4961) (17.0634, 25.3255) (16.896, 25.1706) (16.7989, 25.0623) (16.7654, 25.0108) (16.7397, 24.956) (16.7227, 24.9025) (16.7129, 24.8521) (16.7088, 24.8054) (16.7088, 24.7623) (16.712, 24.7226) (16.7175, 24.6858) (16.7248, 24.6513) (16.7336, 24.6187) (16.7436, 24.5875) (16.7547, 24.5575) (16.7668, 24.5283) (16.7799, 24.4997) (16.7939, 24.4714) (16.8088, 24.4435) (16.8247, 24.4156) (16.8416, 24.3878) (16.8594, 24.3599) (16.8783, 24.3319) (16.8981, 24.3037) (16.919, 24.2754) (16.9408, 24.2467) (16.9638, 24.2178) (16.9989, 24.1752) (17.0375, 24.1305) (17.0784, 24.0781) (17.1142, 24.0305) (17.1553, 23.9733) (17.2013, 23.9063) (17.2519, 23.8294) (17.3066, 23.7422) (17.3651, 23.6446) (17.4268, 23.5363) (17.4915, 23.4173) (17.5586, 23.2874) (17.6277, 23.1463) (17.6985, 22.994) (17.8255, 22.7046) (17.9195, 22.462) (17.9865, 22.2731) knots 0 0 0 0 0.085622 0.111078 0.134991 0.157361 0.178189 0.197474 0.215216 0.231415 0.246072 0.259186 0.270757 0.280785 0.28927 0.296213 0.309142 0.314525 0.319779 0.32491 0.329923 0.334826 0.339627 0.344336 0.348964 0.353525 0.358035 0.362514 0.366985 0.371475 0.37602 0.380661 0.385447 0.39044 0.395711 0.401345 0.407436 0.41408 0.421363 0.429333 0.437971 0.447155 0.455484 0.5 0.544516 0.552845 0.562029 0.570667 0.578637 0.58592 0.592564 0.598655 0.604289 0.60956 0.614553 0.619339 0.62398 0.628525 0.633015 0.637486 0.641965 0.646475 0.651036 0.655664 0.660373 0.665174 0.670077 0.67509 0.680221 0.685475 0.690858 0.703787 0.71073 0.719215 0.729243 0.740814 0.753928 0.768585 0.784784 0.802526 0.821811 0.842639 0.865009 0.888922 0.914378 1 1 1 1
  arc A325 (20.1342, 24.4653) -> (20.8519, 25.3233) centre (0.0409, 42.0024) ccw
  spline S121 degree 3 poles (22.6302, 27.8245) (22.4324, 27.8571) (22.177, 27.9067) (21.8698, 27.9806) (21.7074, 28.0233) (21.5563, 28.0665) (21.4165, 28.1096) (21.2879, 28.1522) (21.1705, 28.1938) (21.0641, 28.2341) (20.9686, 28.2726) (20.8839, 28.3088) (20.8099, 28.3423) (20.7463, 28.3726) (20.6931, 28.3994) (20.6344, 28.4304) (20.5835, 28.4605) (20.5354, 28.4875) (20.5029, 28.505) (20.4708, 28.5215) (20.4392, 28.537) (20.408, 28.5516) (20.3771, 28.5651) (20.3465, 28.5778) (20.3161, 28.5895) (20.2859, 28.6002) (20.2557, 28.61) (20.2255, 28.6188) (20.195, 28.6266) (20.1641, 28.6334) (20.1326, 28.639) (20.1001, 28.6433) (20.0665, 28.6462) (20.0313, 28.6473) (19.994, 28.6462) (19.9544, 28.6423) (19.912, 28.6347) (19.8668, 28.6224) (19.8188, 28.6039) (19.7692, 28.5777) (19.7198, 28.5428) (19.675, 28.5006) (19.5856, 28.386) (19.4627, 28.1938) (19.3215, 28.0146) (19.2426, 27.8924) (19.2175, 27.8363) (19.2007, 27.7781) (19.1923, 27.7227) (19.1906, 27.6713) (19.1938, 27.6245) (19.2006, 27.582) (19.2099, 27.5433) (19.2211, 27.5078) (19.2337, 27.4749) (19.2475, 27.444) (19.2622, 27.4148) (19.2779, 27.3869) (19.2944, 27.3599) (19.3118, 27.3337) (19.3301, 27.308) (19.3492, 27.2827) (19.3693, 27.2577) (19.3903, 27.2329) (19.4123, 27.2081) (19.4352, 27.1834) (19.4592, 27.1587) (19.4843, 27.1339) (19.5104, 27.109) (19.5376, 27.0841) (19.5789, 27.0475) (19.6241, 27.0094) (19.6726, 26.964) (19.7154, 26.9226) (19.7649, 26.8725) (19.8209, 26.8136) (19.8829, 26.7455) (19.9506, 26.6679) (20.0236, 26.5807) (20.1015, 26.4835) (20.184, 26.376) (20.2706, 26.2581) (20.361, 26.1296) (20.4547, 25.9902) (20.6254, 25.7243) (20.7561, 25.4994) (20.8519, 25.3233) knots 0 0 0 0 0.085622 0.111078 0.134991 0.157361 0.178189 0.197474 0.215216 0.231415 0.246072 0.259186 0.270757 0.280785 0.28927 0.296213 0.309142 0.314525 0.319779 0.32491 0.329923 0.334826 0.339627 0.344336 0.348964 0.353525 0.358035 0.362514 0.366985 0.371475 0.37602 0.380661 0.385447 0.39044 0.395711 0.401345 0.407436 0.41408 0.421363 0.429333 0.437971 0.447155 0.455484 0.5 0.544516 0.552845 0.562029 0.570667 0.578637 0.58592 0.592564 0.598655 0.604289 0.60956 0.614553 0.619339 0.62398 0.628525 0.633015 0.637486 0.641965 0.646475 0.651036 0.655664 0.660373 0.665174 0.670077 0.67509 0.680221 0.685475 0.690858 0.703787 0.71073 0.719215 0.729243 0.740814 0.753928 0.768585 0.784784 0.802526 0.821811 0.842639 0.865009 0.888922 0.914378 1 1 1 1
  arc A326 (22.6302, 27.8245) -> (23.2048, 28.7842) centre (0.0409, 42.0024) ccw
  spline S122 degree 3 poles (24.57, 31.5328) (24.3696, 31.534) (24.1096, 31.5431) (23.7945, 31.568) (23.6274, 31.5848) (23.4715, 31.6038) (23.3267, 31.6245) (23.193, 31.6465) (23.0705, 31.6693) (22.9591, 31.6924) (22.8588, 31.7154) (22.7695, 31.7379) (22.6911, 31.7594) (22.6236, 31.7795) (22.5668, 31.7976) (22.504, 31.819) (22.449, 31.8408) (22.3973, 31.86) (22.3624, 31.8722) (22.3282, 31.8834) (22.2945, 31.8938) (22.2614, 31.9033) (22.2288, 31.9119) (22.1966, 31.9195) (22.1648, 31.9263) (22.1332, 31.9322) (22.1019, 31.9372) (22.0706, 31.9411) (22.0393, 31.9441) (22.0077, 31.9459) (21.9757, 31.9465) (21.943, 31.9458) (21.9093, 31.9433) (21.8744, 31.9389) (21.8378, 31.932) (21.7992, 31.9219) (21.7585, 31.9078) (21.7158, 31.8886) (21.6713, 31.8628) (21.6264, 31.8292) (21.5831, 31.7869) (21.5454, 31.7383) (21.4751, 31.6111) (21.3837, 31.402) (21.2723, 31.2029) (21.2135, 31.07) (21.1975, 31.0106) (21.19, 30.9505) (21.1904, 30.8944) (21.1967, 30.8434) (21.2072, 30.7977) (21.2205, 30.7568) (21.2358, 30.72) (21.2524, 30.6867) (21.27, 30.6561) (21.2884, 30.6278) (21.3076, 30.6013) (21.3274, 30.5762) (21.3479, 30.5521) (21.3692, 30.5289) (21.3913, 30.5064) (21.4142, 30.4844) (21.4379, 30.4629) (21.4625, 30.4416) (21.4881, 30.4206) (21.5147, 30.3998) (21.5422, 30.3791) (21.5708, 30.3586) (21.6005, 30.3381) (21.6313, 30.3177) (21.6778, 30.288) (21.7284, 30.2574) (21.7834, 30.2203) (21.8322, 30.186) (21.8889, 30.1443) (21.9534, 30.0949) (22.0253, 30.0373) (22.1043, 29.9713) (22.19, 29.8965) (22.2822, 29.8127) (22.3805, 29.7195) (22.4845, 29.6166) (22.5938, 29.5038) (22.7082, 29.3808) (22.9184, 29.1449) (23.0827, 28.9431) (23.2048, 28.7842) knots 0 0 0 0 0.085622 0.111078 0.134991 0.157361 0.178189 0.197474 0.215216 0.231415 0.246072 0.259186 0.270757 0.280785 0.28927 0.296213 0.309142 0.314525 0.319779 0.32491 0.329923 0.334826 0.339627 0.344336 0.348964 0.353525 0.358035 0.362514 0.366985 0.371475 0.37602 0.380661 0.385447 0.39044 0.395711 0.401345 0.407436 0.41408 0.421363 0.429333 0.437971 0.447155 0.455484 0.5 0.544516 0.552845 0.562029 0.570667 0.578637 0.58592 0.592564 0.598655 0.604289 0.60956 0.614553 0.619339 0.62398 0.628525 0.633015 0.637486 0.641965 0.646475 0.651036 0.655664 0.660373 0.665174 0.670077 0.67509 0.680221 0.685475 0.690858 0.703787 0.71073 0.719215 0.729243 0.740814 0.753928 0.768585 0.784784 0.802526 0.821811 0.842639 0.865009 0.888922 0.914378 1 1 1 1
  arc A327 (24.57, 31.5328) -> (24.9874, 32.5705) centre (0.0409, 42.0024) ccw
  spline S123 degree 3 poles (25.9058, 35.4989) (25.7077, 35.4688) (25.4494, 35.437) (25.1344, 35.4124) (24.9667, 35.4028) (24.8097, 35.3972) (24.6634, 35.395) (24.528, 35.3957) (24.4034, 35.3991) (24.2898, 35.4045) (24.1871, 35.4116) (24.0954, 35.4198) (24.0146, 35.4288) (23.9448, 35.438) (23.8859, 35.4471) (23.8204, 35.4584) (23.7628, 35.4713) (23.7087, 35.4822) (23.6723, 35.4887) (23.6367, 35.4945) (23.6019, 35.4995) (23.5677, 35.5037) (23.5341, 35.507) (23.5011, 35.5096) (23.4686, 35.5113) (23.4366, 35.5122) (23.4048, 35.5122) (23.3733, 35.5112) (23.3419, 35.5092) (23.3105, 35.5061) (23.2787, 35.5017) (23.2466, 35.4958) (23.2137, 35.4881) (23.1798, 35.4783) (23.1448, 35.4658) (23.1083, 35.4498) (23.0703, 35.4295) (23.0311, 35.4038) (22.9912, 35.3714) (22.9521, 35.3312) (22.9159, 35.2826) (22.8863, 35.2287) (22.8367, 35.092) (22.7792, 34.8713) (22.7004, 34.6572) (22.663, 34.5167) (22.6565, 34.4555) (22.6585, 34.395) (22.6677, 34.3397) (22.6819, 34.2903) (22.6994, 34.2468) (22.719, 34.2084) (22.7398, 34.1745) (22.7614, 34.1442) (22.7836, 34.1168) (22.8062, 34.0917) (22.8293, 34.0685) (22.8528, 34.0468) (22.8768, 34.0262) (22.9015, 34.0067) (22.9268, 33.9879) (22.9528, 33.9698) (22.9796, 33.9522) (23.0073, 33.935) (23.0358, 33.9183) (23.0653, 33.9019) (23.0958, 33.8858) (23.1273, 33.87) (23.1598, 33.8544) (23.1933, 33.839) (23.2439, 33.817) (23.2987, 33.7947) (23.3588, 33.7666) (23.4124, 33.7404) (23.475, 33.7081) (23.5464, 33.6694) (23.6264, 33.6237) (23.7147, 33.5709) (23.8111, 33.5105) (23.9153, 33.4421) (24.0269, 33.3654) (24.1457, 33.28) (24.2714, 33.1857) (24.4036, 33.0821) (24.6481, 32.882) (24.842, 32.7085) (24.9874, 32.5705) knots 0 0 0 0 0.085622 0.111078 0.134991 0.157361 0.178189 0.197474 0.215216 0.231415 0.246072 0.259186 0.270757 0.280785 0.28927 0.296213 0.309142 0.314525 0.319779 0.32491 0.329923 0.334826 0.339627 0.344336 0.348964 0.353525 0.358035 0.362514 0.366985 0.371475 0.37602 0.380661 0.385447 0.39044 0.395711 0.401345 0.407436 0.41408 0.421363 0.429333 0.437971 0.447155 0.455484 0.5 0.544516 0.552845 0.562029 0.570667 0.578637 0.58592 0.592564 0.598655 0.604289 0.60956 0.614553 0.619339 0.62398 0.628525 0.633015 0.637486 0.641965 0.646475 0.651036 0.655664 0.660373 0.665174 0.670077 0.67509 0.680221 0.685475 0.690858 0.703787 0.71073 0.719215 0.729243 0.740814 0.753928 0.768585 0.784784 0.802526 0.821811 0.842639 0.865009 0.888922 0.914378 1 1 1 1
  circle A328 centre (0.0409, 42.0024) radius 8.89
  arc A329 (-22.225, 12.7) -> (-28.575, 6.35) centre (-22.225, 6.35) ccw
  line L68 (-28.575, 6.35) -> (-28.575, -6.35)
  arc A330 (-28.575, -6.35) -> (-22.225, -12.7) centre (-22.225, -6.35) ccw
  line L69 (-22.225, -12.7) -> (22.225, -12.7)
  arc A331 (22.225, -12.7) -> (28.575, -6.35) centre (22.225, -6.35) ccw
  line L70 (28.575, -6.35) -> (28.575, 6.35)
  arc A332 (28.575, 6.35) -> (22.225, 12.7) centre (22.225, 6.35) ccw
  line L71 (22.225, 12.7) -> (-22.225, 12.7)
  circle A333 centre (23.8125, 0) radius 2.4892
  circle A334 centre (-23.8125, 0) radius 2.4892
  arc A335 (7.0871, -0.8975) -> (7.0871, 0.8975) centre (7.4422, 0) ccw
  arc A336 (-7.0871, -0.8975) -> (7.0871, -0.8975) centre (0, 0) ccw
  arc A337 (-7.0871, 0.8975) -> (-7.0871, -0.8975) centre (-7.4422, 0) ccw
  arc A338 (7.0871, 0.8975) -> (-7.0871, 0.8975) centre (0, 0) ccw
  line L72 (-48.9582, -13.9669) -> (-18.6452, -31.7617)
  arc A339 (-18.6452, -31.7617) -> (18.6452, -31.7617) centre (0, 0) ccw
  line L73 (18.6452, -31.7617) -> (56.4257, -9.5833)
  arc A340 (56.4257, -9.5833) -> (61.6428, -2.4333) centre (50.8, 0) ccw
  line L74 (61.6428, -2.4333) -> (77.754, 69.3573)
  arc A341 (77.754, 69.3573) -> (75.8031, 89.663) centre (45.7832, 76.5321) ccw
  line L75 (69.2061, 99.4446) -> (35.9152, 133.5377)
  line L76 (-35.8282, 133.6268) -> (-69.207, 99.4446)
  arc A342 (35.9152, 133.5377) -> (-35.8282, 133.6268) centre (-0.0477, 60.1323) ccw
  arc A343 (-69.207, 99.4446) -> (-45.7832, 32.916) centre (28.0956, 96.3156) ccw
  arc A344 (-45.7832, 32.916) -> (0.0538, 13.3581) centre (-4.4276, 66.3474) ccw
  line L77 (-45.7832, 32.916) -> (94.2389, 32.916) construction
  line L78 (-69.207, 99.4446) -> (69.2061, 99.4446) construction
  arc A345 (0.0538, 13.3581) -> (45.8908, 32.916) centre (4.5351, 66.3474) ccw
  arc A346 (45.8908, 32.916) -> (69.2061, 99.4446) centre (-28.0925, 96.1937) ccw
  line L79 (-34.8862, 132.3193) -> (-67.6381, 98.779)
  arc A347 (-67.6381, 98.779) -> (-44.5633, 33.9321) centre (28.0956, 96.3156) ccw
  arc A348 (-44.5633, 33.9321) -> (0.0538, 14.9514) centre (-4.4276, 66.3474) ccw
  arc A349 (0.0538, 14.9514) -> (44.67, 33.9311) centre (4.5351, 66.3474) ccw
  arc A350 (44.67, 33.9311) -> (67.638, 98.7782) centre (-28.0925, 96.1937) ccw
  line L80 (67.638, 98.7782) -> (34.9717, 132.2316)
  arc A351 (34.9717, 132.2316) -> (-34.8862, 132.3193) centre (-0.0477, 60.1323) ccw
  point P0 (0.0538, 15.3324)
  dimension "d0" = 2.6324
  dimension "d1" = 0.6581
  dimension "d2" = 45.837
  dimension "d3" = 45.837
  dimension "d4" = 53.1784
  dimension "d5" = 53.1784
  dimension "d6" = 97.3529
  dimension "d7" = 97.3529
  dimension "d8" = 1.5875
  constraints: 26 point on circle, 18 end point, 13 centre point, 3 point on line, 2 horizontal, 9 other
  measures "d0" distance from line of L71 point (0.054, 15.332)
  measures "d1" distance from line of L71 A344.end
  measures "d2" horizontal distance of L77.start A344.end
  measures "d3" horizontal distance of A344.end A345.end
  measures "d4" radius of A344
  measures "d5" radius of A345
  measures "d6" radius of A346
  measures "d7" radius of A343
  measures "d8" radial gap between concentric circles of A342 A351
extrude "Extrusion1" add sketch "Sketch1" along normal blind 38.1 contours L5 A342 L45 A351 L79 A347 A131 A343 | A131 A347 L42 A343 | A342 L46 A142 A351 L45 | L42 A347 L22 A343 | A342 L60 A185 A351 A142 L46 | L22 A347 L24 A343 | L4 A346 A20 A350 L80 A351 L61 A342 | A342 L61 A351 A185 L60 | L24 A347 L31 A343 | L31 A347 A348 L33 A344 A343 | A346 L8 A350 A20 | A346 L47 A350 L8 | L33 A348 L30 A344 | A346 L49 A350 L47 | L30 A348 A89 A90 A91 A344 | A346 L9 A350 L49 | A91 A90 A89 A348 A349 A155 A154 A153 A345 A9 A344 | A346 A345 L11 A349 A350 L9 | A9 A345 A344 | A345 L51 A349 L11 | A349 L51 A345 A153 A154 A155
sketch "Sketch2" plane through (0, 0, 38.1) normal (0, 0, 1) x (1, 0, 0)
  line L0 (-35.8282, 133.6268) -> (-69.207, 99.4446) projected
  arc A0 (35.9152, 133.5377) -> (-35.8282, 133.6268) centre (-0.0477, 60.1323) ccw projected
  line L1 (69.2061, 99.4446) -> (35.9152, 133.5377) projected
  arc A1 (45.8908, 32.916) -> (69.2061, 99.4446) centre (-28.0925, 96.1937) ccw projected
  arc A2 (0.0538, 13.3581) -> (45.8908, 32.916) centre (4.5351, 66.3474) ccw projected
  arc A3 (-45.7832, 32.916) -> (0.0538, 13.3581) centre (-4.4276, 66.3474) ccw projected
  arc A4 (-69.207, 99.4446) -> (-45.7832, 32.916) centre (28.0956, 96.3156) ccw projected
  line L2 (-69.207, 99.4446) -> (-35.8282, 133.6268)
  arc A5 (35.9152, 133.5377) -> (-35.8282, 133.6268) centre (-0.0477, 60.1323) ccw
  line L3 (35.9152, 133.5377) -> (69.2061, 99.4446)
  arc A6 (45.8908, 32.916) -> (69.2061, 99.4446) centre (-28.0925, 96.1937) ccw
  arc A7 (0.0538, 13.3581) -> (45.8908, 32.916) centre (4.5351, 66.3474) ccw
  arc A8 (-45.7832, 32.916) -> (0.0538, 13.3581) centre (-4.4276, 66.3474) ccw
  arc A9 (-69.207, 99.4446) -> (-45.7832, 32.916) centre (28.0956, 96.3156) ccw
  point P0 (0, 0)
  constraints: 10 point on circle, 5 centre point, 4 end point, 6 other
extrude "Extrusion2" add sketch "Sketch2" along normal blind 1.5875
sketch "Sketch3" plane through (0, 0, 39.6875) normal (0, 0, 1) x (1, 0, 0)
  line L0 (-69.207, 99.4446) -> (-35.8282, 133.6268) projected
  arc A0 (-69.207, 99.4446) -> (-45.7832, 32.916) centre (28.0956, 96.3156) ccw projected
  arc A1 (-45.7832, 32.916) -> (0.0538, 13.3581) centre (-4.4276, 66.3474) ccw projected
  arc A2 (0.0538, 13.3581) -> (45.8908, 32.916) centre (4.5351, 66.3474) ccw projected
  arc A3 (45.8908, 32.916) -> (69.2061, 99.4446) centre (-28.0925, 96.1937) ccw projected
  line L1 (35.9152, 133.5377) -> (69.2061, 99.4446) projected
  arc A4 (35.9152, 133.5377) -> (-35.8282, 133.6268) centre (-0.0477, 60.1323) ccw projected
  circle A5 centre (45.7832, 101.9321) radius 3.4798 projected
  arc A6 (48.0396, 102.3311) -> (46.5659, 104.0857) centre (45.7832, 101.9321) ccw projected
  arc A7 (47.2569, 100.1775) -> (48.0396, 102.3311) centre (45.7832, 101.9321) ccw projected
  arc A8 (45.0005, 99.7786) -> (47.2569, 100.1775) centre (45.7832, 101.9321) ccw projected
  arc A9 (43.5269, 101.5332) -> (45.0005, 99.7786) centre (45.7832, 101.9321) ccw projected
  arc A10 (44.3096, 103.6868) -> (43.5269, 101.5332) centre (45.7832, 101.9321) ccw projected
  arc A11 (46.5659, 104.0857) -> (44.3096, 103.6868) centre (45.7832, 101.9321) ccw projected
  circle A12 centre (45.7832, 51.1321) radius 3.4798 projected
  arc A13 (48.0387, 51.5361) -> (46.5611, 53.2874) centre (45.7832, 51.1321) ccw projected
  arc A14 (47.2608, 49.3808) -> (48.0387, 51.5361) centre (45.7832, 51.1321) ccw projected
  arc A15 (45.0053, 48.9769) -> (47.2608, 49.3808) centre (45.7832, 51.1321) ccw projected
  arc A16 (43.5278, 50.7282) -> (45.0053, 48.9769) centre (45.7832, 51.1321) ccw projected
  arc A17 (44.3056, 52.8835) -> (43.5278, 50.7282) centre (45.7832, 51.1321) ccw projected
  arc A18 (46.5611, 53.2874) -> (44.3056, 52.8835) centre (45.7832, 51.1321) ccw projected
  circle A19 centre (-45.7832, 51.1321) radius 3.4798 projected
  arc A20 (-45.0442, 48.9632) -> (-43.5354, 50.6877) centre (-45.7832, 51.1321) ccw projected
  arc A21 (-47.292, 49.4077) -> (-45.0442, 48.9632) centre (-45.7832, 51.1321) ccw projected
  arc A22 (-48.0311, 51.5766) -> (-47.292, 49.4077) centre (-45.7832, 51.1321) ccw projected
  arc A23 (-46.5222, 53.3011) -> (-48.0311, 51.5766) centre (-45.7832, 51.1321) ccw projected
  arc A24 (-44.2744, 52.8566) -> (-46.5222, 53.3011) centre (-45.7832, 51.1321) ccw projected
  arc A25 (-43.5354, 50.6877) -> (-44.2744, 52.8566) centre (-45.7832, 51.1321) ccw projected
  circle A26 centre (-45.7832, 101.9321) radius 3.4798 projected
  arc A27 (-43.5256, 102.3238) -> (-44.9936, 104.0831) centre (-45.7832, 101.9321) ccw projected
  arc A28 (-44.3152, 100.1728) -> (-43.5256, 102.3238) centre (-45.7832, 101.9321) ccw projected
  arc A29 (-46.5729, 99.7812) -> (-44.3152, 100.1728) centre (-45.7832, 101.9321) ccw projected
  arc A30 (-48.0409, 101.5405) -> (-46.5729, 99.7812) centre (-45.7832, 101.9321) ccw projected
  arc A31 (-47.2512, 103.6915) -> (-48.0409, 101.5405) centre (-45.7832, 101.9321) ccw projected
  arc A32 (-44.9936, 104.0831) -> (-47.2512, 103.6915) centre (-45.7832, 101.9321) ccw projected
  circle A33 centre (45.7832, 101.9321) radius 4.7625
  circle A34 centre (45.7832, 51.1321) radius 4.7625
  circle A35 centre (-45.7832, 101.9321) radius 4.7625
  circle A36 centre (-45.7832, 51.1321) radius 4.7625
  point P0 (0, 0)
  dimension "d13" = 9.525
  dimension "d14" = 9.525
  dimension "d15" = 9.525
  dimension "d18" = 9.525
  constraints: 4 centre point, 4 coincident
  measures "d13" diameter of A34
  measures "d14" diameter of A35
  measures "d15" diameter of A36
  measures "d18" diameter of A33
sketch "Sketch4" plane through (0, 0, 0) normal (1, 0, 0) x (0, 1, 0)
  line L0 (15.8875, 10.9721) -> (15.8875, 1.4471) projected
  line L1 (47.1697, 36.0934) -> (47.1697, 31.9913)
  line L2 (47.1697, 36.0934) -> (47.1697, 31.9913)
  line L3 (54.6119, 36.576) -> (47.6523, 36.576) projected
  line L4 (32.916, 0) -> (13.3581, 0) projected
  line L5 (32.916, 0) -> (32.916, 39.6875) projected
  line L6 (13.1689, 39.6875) -> (13.3581, 39.6875) projected
  line L7 (13.3581, 0) -> (13.3581, 39.6875) projected
  line L8 (99.4446, 0) -> (32.916, 0) projected
  line L9 (99.4446, 0) -> (99.4446, 39.6875) projected
  line L10 (32.916, 39.6875) -> (32.916, 39.6875) projected
  line L11 (32.916, 0) -> (32.916, 39.6875) projected
  line L12 (13.1689, 39.6875) -> (32.916, 39.6875) projected
  line L13 (46.3457, 39.6875) -> (13.1689, 12.4876)
  line L14 (13.1689, 0) -> (13.1689, 39.6875) projected
  line L15 (13.3581, 10.5899) -> (48.8496, 39.6875)
  line L16 (13.3581, 10.5899) -> (13.1689, 10.5036)
  line L17 (13.1689, 10.5036) -> (13.1689, 12.4876)
  line L18 (48.8496, 39.6875) -> (46.3457, 39.6875)
  line L19 (46.3457, 39.6875) -> (13.1689, 39.6875)
  line L20 (13.1689, 39.6875) -> (13.1689, 12.4876)
  point P0 (0, 0)
  dimension "d19" = 1.5875
  constraints: 18 end point, 3 point on line, 2 collinear, 2 parallel, 2 vertical, 1 perpendicular, 2 other
  measures "d19" distance between parallel lines of L13 L15
extrude "Extrusion4" cut sketch "Sketch4" along normal through all both and the other way through all contours L15 L7 L13 L5 | L5 L13 L18 L15 | L16 L14 L13 L7 | L13 L7 L12 L5 | L5 L19 L13 | L13 L14 L6 L7
sketch "Sketch6" plane through (0, 0, 0) normal (1, 0, 0) x (0, 1, 0)
  line L0 (32.916, 26.6244) -> (48.8496, 39.6875) projected
  line L1 (13.3581, 10.5899) -> (32.916, 26.6244) projected
  line L2 (13.3581, 10.5899) -> (32.916, 26.6244) projected
  line L3 (48.8496, 39.6875) -> (13.3581, 10.5899)
  line L4 (13.3581, 10.5899) -> (13.3581, 12.6427)
  line L5 (13.3581, 12.6427) -> (46.3457, 39.6875)
  line L6 (46.3457, 39.6875) -> (48.8496, 39.6875)
  point P0 (0, 0)
  dimension "d22" = 1.5875
  constraints: 8 end point, 2 parallel, 1 collinear, 1 perpendicular, 1 vertical
  measures "d22" distance between parallel lines of L5 L0
extrude "Extrusion5" add sketch "Sketch6" along normal mid plane 127
sketch "Sketch8" plane through (0, 0, 39.6875) normal (0, 0, 1) x (1, 0, 0)
  arc A0 (-56.9018, 48.8496) -> (-45.7832, 32.916) centre (28.0956, 96.3156) ccw projected
  arc A1 (-45.7832, 32.916) -> (-8.9089, 13.3581) centre (-4.4276, 66.3474) ccw projected
  arc A2 (45.8908, 32.916) -> (56.9729, 48.8496) centre (-28.0925, 96.1937) ccw projected
  arc A3 (9.0165, 13.3581) -> (45.8908, 32.916) centre (4.5351, 66.3474) ccw projected
  line L0 (-8.9089, 13.3581) -> (9.0165, 13.3581)
  line L1 (-63.5, 13.3581) -> (63.5, 13.3581) projected
  line L2 (-56.9018, 48.8496) -> (-63.5, 48.8496) projected
  line L3 (-56.9018, 48.8496) -> (-63.5, 48.8496)
  line L4 (-63.5, 48.8496) -> (-63.5, 13.3581)
  line L5 (-63.5, 13.3581) -> (-8.9089, 13.3581)
  line L6 (9.0165, 13.3581) -> (66.4862, 13.3581)
  line L7 (66.4862, 13.3581) -> (66.4862, 48.8496)
  line L8 (63.5, 48.8496) -> (56.9729, 48.8496) projected
  line L9 (66.4862, 48.8496) -> (56.9729, 48.8496)
  point P0 (0, 0)
  constraints: 14 end point, 4 perpendicular, 3 point on line, 2 collinear
extrude "Extrusion6" cut sketch "Sketch8" against normal through all